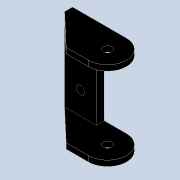
# Autodesk Inventor part: Y Axis Drag Chain Mount Stationary
Saved by Autodesk Inventor 2022 (Build 260153000, 153)
## iProperties
Created: 2021-10-30
Part Number: Y Axis Drag Chain Mount Stationary
Material: Generic
Document SubType Name: Modeling
Designer: Coy
Density: 1 g/cm^3
Appearance: Anodized - Black
Author: Coy
Autodesk Inventor part; units mm, degrees
ref_plane "YZ Plane" through (0, 0, 0) normal (1, 0, 0) x (0, 1, 0)
ref_plane "XZ Plane" through (0, 0, 0) normal (0, 1, 0) x (-1, 0, 0)
ref_plane "XY Plane" through (0, 0, 0) normal (0, 0, 1) x (1, 0, 0)
sketch "Sketch1" plane through (0, 0, 0) normal (0, 0, 1) x (1, 0, 0)
  line L0 (0, 0) -> (-20, 0)
  line L1 (-20, 0) -> (-20, 55.5)
  line L2 (-20, 55.5) -> (0, 55.5)
  line L3 (0, 55.5) -> (0, 0)
  line L4 (-10, 0) -> (-10, 55.5) construction
  circle A0 centre (-10, 37.75) radius 2.6
  circle A1 centre (-10, 17.75) radius 2.6
  dimension "d0" = 20
  dimension "d1" = 55.5
  dimension "d2" = 5.2
  dimension "d3" = 5.2
  dimension "d4" = 17.75
  dimension "d5" = 17.75
  constraints: 10 end point, 2 centre point, 2 midpoint, 2 parallel, 2 point on line, 1 horizontal, 1 perpendicular
  measures "d0" distance of L1.end L2.end
  measures "d1" distance of L0.end L1.end
  measures "d2" diameter of A0
  measures "d3" diameter of A1
  measures "d4" distance from line of L2 A0.centre
  measures "d5" distance from line of L0 A1.centre
extrude "Extrusion1" add sketch "Sketch1" along normal blind 5
sketch "Sketch2" plane through (0, 0, 0) normal (1, 0, 0) x (0, 0, -1)
  line L0 (0, 55.5) -> (-5, 55.5) projected
  line L1 (0, 55.5) -> (-24, 55.5)
  line L2 (-24, 55.5) -> (-24, 52)
  line L3 (-24, 52) -> (0, 52)
  line L4 (0, 52) -> (0, 55.5)
  line L5 (0, 0) -> (-5, 0) projected
  line L6 (0, 0) -> (-24, 0)
  line L7 (-24, 0) -> (-24, 3.5)
  line L8 (-24, 3.5) -> (0, 3.5)
  line L9 (0, 3.5) -> (0, 0)
  dimension "d8" = 24
  dimension "d9" = 3.5
  dimension "d10" = 24
  dimension "d11" = 3.5
  constraints: 16 end point, 4 parallel, 2 horizontal, 2 perpendicular
  measures "d8" distance of L3.end L2.end
  measures "d9" distance of L2.end L1.end
  measures "d10" distance of L7.end L8.end
  measures "d11" distance of L6.end L7.end
extrude "Extrusion2" add sketch "Sketch2" along normal blind 26
fillet "Fillet1" radius 12 4 edges at (26, 53.75, 0) (26, 53.75, 24) (26, 1.75, 0) (26, 1.75, 24)
sketch "Sketch3" plane through (-20, 55.5, 5) normal (0, 1, 0) x (1, 0, 0)
  arc A0 (34, -19) -> (34, 5) centre (34, -7) ccw projected
  circle A1 centre (34, -7) radius 2.75
  point P0 (20, 5)
  dimension "d15" = 5.5
  constraints: 1 centre point, 1 coincident
  measures "d15" diameter of A1
extrude "Extrusion3" cut sketch "Sketch3" against normal through all
chamfer "Chamfer1" distance 20 distance2 19 1 edges at (0, 53.75, 5) measured on face at (-17.5081, 30.8759, 5)
chamfer "Chamfer2" distance 20 distance2 19 1 edges at (0, 1.75, 5) measured on face at (-17.508, 23.4574, 5)
equation "\"d3\" = d2"
equation "\"d5\" = d4"
body "Solid1"
